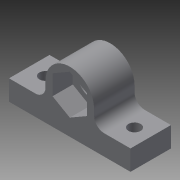
# Autodesk Inventor part: motor_bracket
Saved by Autodesk Inventor 2015 (Build 190159000, 159)
## iProperties
Created: 2015-12-01
Part Number: motor_bracket
Material: Generic
Document SubType Name: Modeling
Designer: jufranz
Density: 1 g/cm^3
Appearance: Default
Author: jufranz
Autodesk Inventor part; units mm, degrees
ref_plane "YZ Plane" through (0, 0, 0) normal (1, 0, 0) x (0, 1, 0)
ref_plane "XZ Plane" through (0, 0, 0) normal (0, 1, 0) x (-1, 0, 0)
ref_plane "XY Plane" through (0, 0, 0) normal (0, 0, 1) x (1, 0, 0)
sketch "Sketch1" plane through (0, 0, 0) normal (0, 1, 0) x (-1, 0, 0)
  line L0 (15, 5) -> (-15, 5)
  line L1 (-15, 5) -> (-15, -5)
  line L2 (-15, -5) -> (15, -5)
  line L3 (15, -5) -> (15, 5)
  point P0 (0, 0)
  point P1 (15, 0)
  point P2 (0, 5)
  dimension "d0" = 30
  dimension "d1" = 10
  constraints: 8 end point, 2 midpoint, 2 parallel, 1 horizontal, 1 horizontal alignment, 1 perpendicular, 1 vertical alignment
  measures "d0" distance of L0.start L0.end
  measures "d1" distance between parallel lines of L2 L0
extrude "Extrusion1" add sketch "Sketch1" along normal blind 5
sketch "Sketch3" plane through (0, 5, 0) normal (0, 1, 0) x (1, 0, 0)
  line L0 (-15, -5) -> (15, -5) projected
  line L1 (-6, 5) -> (6, 5)
  line L2 (6, 5) -> (6, -5)
  line L3 (6, -5) -> (-6, -5)
  line L4 (-6, -5) -> (-6, 5)
  line L5 (15, 5) -> (-15, 5) projected
  point P0 (0, 0)
  point P1 (0, 5)
  dimension "d13" = 12
  dimension "d14" = 6
  constraints: 8 end point, 2 midpoint, 2 parallel, 1 horizontal, 1 perpendicular, 1 point on line
  measures "d13" distance between parallel lines of L4 L2
  measures "d14" distance from line of L4 point (0, 0)
extrude "Extrusion2" add sketch "Sketch3" along normal blind 10
sketch "Sketch4" plane through (-15, 0, 5) normal (0, 0, 1) x (1, 0, 0)
  line L0 (9, 15) -> (21, 15) projected
  line L1 (9, 5) -> (9, 15) projected
  line L2 (0, 5) -> (9, 5) projected
  point P0 (15, 0)
  point P1 (15, 9)
  dimension "d18" = 6
  dimension "d43" = 4
  measures "d18" distance from line of L1 point (15, 9)
  measures "d43" distance from line of L2 point (15, 9)
hole "Hole2" at (0, 9, 5) direction (0, 0, -1) diameter 6 end through all
sketch "Sketch5" plane through (-15, 0, 5) normal (0, 0, 1) x (1, 0, 0)
  line L0 (15, 4.0925) -> (10.75, 6.5463)
  line L1 (10.75, 6.5463) -> (10.75, 11.4537)
  line L2 (10.75, 11.4537) -> (15, 13.9075)
  line L3 (15, 13.9075) -> (19.25, 11.4537)
  line L4 (19.25, 11.4537) -> (19.25, 6.5463)
  line L5 (19.25, 6.5463) -> (15, 4.0925)
  line L6 (9, 15) -> (21, 15) projected
  line L7 (21, 5) -> (21, 15) projected
  line L8 (0, 5) -> (9, 5) projected
  point P0 (15, 0)
  point P1 (15, 9)
  point P2 (13.175, 20)
  point P3 (16.825, 20)
  point P4 (20, 13.175)
  point P5 (20, 16.825)
  dimension "d28" = 6
  dimension "d42" = 8.5
  dimension "d44" = 4
  constraints: 12 end point, 1 vertical alignment, 15 other
  measures "d42" distance between parallel lines of L4 L1
  measures "d44" distance from line of L8 point (15, 9)
extrude "Extrusion3" cut sketch "Sketch5" against normal blind 5
fillet "Fillet2" radius 6 2 edges at (-6, 15, 0) (6, 15, 0)
fillet "Fillet3" radius 2.5 2 edges at (6, 5, 0) (-6, 5, 0)
sketch "Sketch6" plane through (0, 0, 0) normal (0, -1, 0) x (1, 0, 0)
  line L0 (-15, -5) -> (-15, 5) projected
  line L1 (15, 5) -> (15, -5) projected
  point P0 (0, 0)
  point P1 (-11, 0)
  point P2 (11, 0)
  dimension "d33" = 4
  dimension "d34" = 4
  constraints: 2 horizontal alignment
  measures "d33" distance from line of L0 point (-11, 0)
  measures "d34" distance from line of L1 point (11, 0)
hole "Hole3" at (-11, 0, 0) at (11, 0, 0) direction (0, 1, 0) diameter 3 end through all
equation "\"d14\" = 0.5 * d13"
equation "\"d18\" = d17"
equation "\"d44\" = d43"
equation "\"d34\" = d33"
equation "\"d17\" = 6"
body "Solid1"
